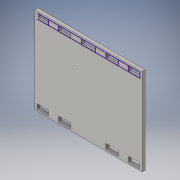
# Autodesk Inventor part: mcdave_scelevel
Saved by Autodesk Inventor 2016 (Build 200138000, 138)
## iProperties
Created: 2017-11-27
Part Number: mcdave_scelevel
Material: Generic
Document SubType Name: Modeling
Designer: student
Density: 1 g/cm^3
Appearance: Default
Author: student
Autodesk Inventor part; units mm, degrees
ref_plane "YZ Plane" through (0, 0, 0) normal (1, 0, 0) x (0, 1, 0)
ref_plane "XZ Plane" through (0, 0, 0) normal (0, 1, 0) x (-1, 0, 0)
ref_plane "XY Plane" through (0, 0, 0) normal (0, 0, 1) x (1, 0, 0)
sketch "Sketch1" plane through (0, 0, 0) normal (0, 0, 1) x (1, 0, 0)
  line L0 (49.1624, -46.1074) -> (-32.1176, -46.1074)
  line L1 (49.1624, 19.9326) -> (49.1624, -46.1074)
  line L2 (49.1624, -46.1074) -> (49.1624, 19.9326)
  line L3 (-32.1176, 19.9326) -> (49.1624, 19.9326)
  line L4 (49.1624, 19.9326) -> (-32.1176, 19.9326)
  line L5 (-32.1176, -46.1074) -> (-32.1176, 19.9326)
  line L6 (-32.1176, 19.9326) -> (-32.1176, -46.1074)
  line L7 (-32.1176, -46.1074) -> (49.1624, -46.1074)
  line L8 (47.5774, -44.8414) -> (38.8489, -44.8414)
  line L9 (47.5774, -44.8414) -> (38.8489, -44.8414)
  line L10 (38.8489, -40.9552) -> (38.8489, -44.8414)
  line L11 (38.8489, -44.8414) -> (38.8489, -40.9552)
  line L12 (38.8489, -40.9552) -> (47.5774, -40.9552)
  line L13 (38.8489, -40.9552) -> (47.5774, -40.9552)
  line L14 (47.5774, -40.9552) -> (47.5774, -44.8414)
  line L15 (47.5774, -40.9552) -> (47.5774, -44.8414)
  line L16 (47.5774, 14.7804) -> (38.8489, 14.7804)
  line L17 (47.5774, 14.7804) -> (38.8489, 14.7804)
  line L18 (38.8489, 14.7804) -> (38.8489, 18.6666)
  line L19 (38.8489, 14.7804) -> (38.8489, 18.6666)
  line L20 (38.8489, 18.6666) -> (47.5774, 18.6666)
  line L21 (38.8489, 18.6666) -> (47.5774, 18.6666)
  line L22 (47.5774, 18.6666) -> (47.5774, 14.7804)
  line L23 (47.5774, 18.6666) -> (47.5774, 14.7804)
  line L24 (31.2541, -44.8414) -> (21.8023, -44.8414)
  line L25 (31.2541, -44.8414) -> (21.8023, -44.8414)
  line L26 (21.8023, -40.9552) -> (21.8023, -44.8414)
  line L27 (21.8023, -44.8414) -> (21.8023, -40.9552)
  line L28 (21.8023, -40.9552) -> (31.2541, -40.9552)
  line L29 (31.2541, -40.9552) -> (31.2541, -44.8414)
  line L30 (31.2541, -40.9552) -> (31.2541, -44.8414)
  line L31 (-4.7575, -44.8414) -> (-14.2093, -44.8414)
  line L32 (-4.7575, -44.8414) -> (-14.2093, -44.8414)
  line L33 (-14.2093, -40.9552) -> (-14.2093, -44.8414)
  line L34 (-14.2093, -44.8414) -> (-14.2093, -40.9552)
  line L35 (-4.7575, -40.9552) -> (-14.2093, -40.9552)
  line L36 (-14.2093, -40.9552) -> (-4.7575, -40.9552)
  line L37 (-4.7575, -40.9552) -> (-4.7575, -44.8414)
  line L38 (-4.7575, -40.9552) -> (-4.7575, -44.8414)
  line L39 (-21.804, -40.9552) -> (-21.804, -44.8414)
  line L40 (-30.5326, -44.8414) -> (-21.804, -44.8414)
  line L41 (-21.804, -44.8414) -> (-30.5326, -44.8414)
  line L42 (-30.5326, -44.8414) -> (-30.5326, -40.9552)
  line L43 (-30.5326, -40.9552) -> (-21.804, -40.9552)
  line L44 (-30.5326, -40.9552) -> (-21.804, -40.9552)
  line L45 (-21.804, -40.9552) -> (-21.804, -44.8414)
  line L46 (31.2541, 14.7804) -> (21.8023, 14.7804)
  line L47 (31.2541, 14.7804) -> (21.8023, 14.7804)
  line L48 (21.8023, 14.7804) -> (21.8023, 18.6666)
  line L49 (21.8023, 14.7804) -> (21.8023, 18.6666)
  line L50 (21.8023, 18.6666) -> (31.2541, 18.6666)
  line L51 (21.8023, 18.6666) -> (31.2541, 18.6666)
  line L52 (31.2541, 18.6666) -> (31.2541, 14.7804)
  line L53 (31.2541, 18.6666) -> (31.2541, 14.7804)
  line L54 (3.2185, 14.7804) -> (13.8264, 14.7804)
  line L55 (13.8264, 14.7804) -> (3.2185, 14.7804)
  line L56 (3.2185, 18.6666) -> (3.2185, 14.7804)
  line L57 (3.2185, 14.7804) -> (3.2185, 18.6666)
  line L58 (3.2185, 18.6666) -> (13.8264, 18.6666)
  line L59 (3.2185, 18.6666) -> (13.8264, 18.6666)
  line L60 (13.8264, 14.7804) -> (13.8264, 18.6666)
  line L61 (13.8264, 18.6666) -> (13.8264, 14.7804)
  line L62 (-4.7575, 14.7804) -> (-14.2093, 14.7804)
  line L63 (-4.7575, 14.7804) -> (-14.2093, 14.7804)
  line L64 (-14.2093, 14.7804) -> (-14.2093, 18.6666)
  line L65 (-14.2093, 14.7804) -> (-14.2093, 18.6666)
  line L66 (-14.2093, 18.6666) -> (-4.7575, 18.6666)
  line L67 (-14.2093, 18.6666) -> (-4.7575, 18.6666)
  line L68 (-4.7575, 18.6666) -> (-4.7575, 14.7804)
  line L69 (-4.7575, 18.6666) -> (-4.7575, 14.7804)
  line L70 (-21.804, 18.6666) -> (-21.804, 14.7804)
  line L71 (-21.804, 14.7804) -> (-30.5326, 14.7804)
  line L72 (-21.804, 14.7804) -> (-30.5326, 14.7804)
  line L73 (-30.5326, 18.6666) -> (-21.804, 18.6666)
  line L74 (-30.5326, 14.7804) -> (-30.5326, 18.6666)
  line L75 (-30.5326, 18.6666) -> (-21.804, 18.6666)
  line L76 (-21.804, 18.6666) -> (-21.804, 14.7804)
  point P0 (0, 0)
  point P1 (0, 0)
  constraints: 154 end point, 36 collinear, 4 perpendicular
extrude "Extrusion1" add sketch "Sketch1" along normal blind 2.286
sketch "Sketch2" plane through (0, 0, 2.286) normal (0, 0, 1) x (1, 0, 0)
  line L0 (-30.5326, 18.6666) -> (-30.5326, 14.7804) projected
  line L1 (47.5774, 18.6666) -> (38.8489, 18.6666) projected
  line L2 (-30.5326, 18.6666) -> (47.5774, 18.6666)
  line L3 (47.5774, 18.6666) -> (47.5774, 14.7804) projected
  line L4 (47.5774, 18.6666) -> (47.5774, 14.7804)
  line L5 (-30.5326, 14.7804) -> (-21.804, 14.7804) projected
  line L6 (47.5774, 14.7804) -> (-30.5326, 14.7804)
  line L7 (-21.804, 18.6666) -> (-21.804, 14.7804) projected
  line L8 (-21.804, 18.6666) -> (-21.804, 14.7804)
  line L9 (-4.7575, 18.6666) -> (-14.2093, 18.6666) projected
  line L10 (-14.2093, 14.7804) -> (-14.2093, 18.6666) projected
  line L11 (-14.2093, 18.6666) -> (-14.2093, 14.7804)
  line L12 (3.2185, 14.7804) -> (3.2185, 18.6666) projected
  line L13 (3.2185, 18.6666) -> (3.2185, 14.7804)
  line L14 (13.8264, 18.6666) -> (13.8264, 14.7804) projected
  line L15 (13.8264, 18.6666) -> (13.8264, 14.7804)
  line L16 (21.8023, 18.6666) -> (21.8023, 14.7804)
  line L17 (31.2541, 18.6666) -> (31.2541, 14.7804) projected
  line L18 (31.2541, 18.6666) -> (31.2541, 14.7804)
  line L19 (38.8489, 14.7804) -> (47.5774, 14.7804) projected
  line L20 (38.8489, 18.6666) -> (38.8489, 14.7804)
  point P0 (0, 0)
  constraints: 20 end point, 6 collinear, 3 point on line, 3 vertical, 1 perpendicular
body "Solid1"
